Autodesk Inventor part; units mm, degrees
(part 3 of 3)
  line L755 (119.1, 110.9) -> (119.1, 119.1)
  line L756 (110.9, 100.9) -> (119.1, 100.9)
  line L757 (119.1, 119.1) -> (110.9, 119.1)
  line L758 (110.9, 119.1) -> (110.9, 120.9) construction
  line L759 (110.9, 120.9) -> (119.1, 120.9)
  line L760 (119.1, 120.9) -> (119.1, 129.1)
  line L761 (110.9, 129.1) -> (110.9, 120.9)
  line L762 (119.1, 139.1) -> (110.9, 139.1)
  line L763 (110.9, 140.9) -> (110.9, 139.1) construction
  line L764 (110.9, 130.9) -> (119.1, 130.9)
  line L765 (110.9, 139.1) -> (110.9, 130.9)
  line L766 (119.1, 129.1) -> (110.9, 129.1)
  line L767 (110.9, 129.1) -> (110.9, 130.9) construction
  line L768 (119.1, 130.9) -> (119.1, 139.1)
  line L769 (119.1, 160.9) -> (119.1, 169.1)
  line L770 (110.9, 169.1) -> (110.9, 160.9)
  line L771 (119.1, 169.1) -> (110.9, 169.1)
  line L772 (110.9, 169.1) -> (110.9, 170.9) construction
  line L773 (110.9, 170.9) -> (119.1, 170.9)
  line L774 (110.9, 179.1) -> (110.9, 170.9)
  line L775 (119.1, 170.9) -> (119.1, 179.1)
  line L776 (119.1, 179.1) -> (110.9, 179.1)
  line L777 (119.1, 149.1) -> (110.9, 149.1)
  line L778 (119.1, 140.9) -> (119.1, 149.1)
  line L779 (110.9, 150.9) -> (119.1, 150.9)
  line L780 (110.9, 149.1) -> (110.9, 150.9) construction
  line L781 (119.1, 150.9) -> (119.1, 159.1)
  line L782 (119.1, 159.1) -> (110.9, 159.1)
  line L783 (110.9, 159.1) -> (110.9, 150.9)
  line L784 (110.9, 160.9) -> (119.1, 160.9)
  line L785 (110.9, 159.1) -> (110.9, 160.9) construction
  line L786 (110.9, 149.1) -> (110.9, 140.9)
  line L787 (110.9, 140.9) -> (119.1, 140.9)
  line L788 (119.1, 60.9) -> (119.1, 69.1)
  line L789 (110.9, 69.1) -> (110.9, 60.9)
  line L790 (119.1, 69.1) -> (110.9, 69.1)
  line L791 (110.9, 69.1) -> (110.9, 70.9) construction
  line L792 (110.9, 70.9) -> (119.1, 70.9)
  line L793 (119.1, 70.9) -> (119.1, 79.1)
  line L794 (110.9, 79.1) -> (110.9, 70.9)
  line L795 (119.1, 79.1) -> (110.9, 79.1)
  line L796 (110.9, 79.1) -> (110.9, 80.9) construction
  line L797 (119.1, 80.9) -> (119.1, 89.1)
  line L798 (110.9, 89.1) -> (110.9, 80.9)
  line L799 (110.9, 80.9) -> (119.1, 80.9)
  line L800 (109.1, 20.9) -> (110.9, 20.9) construction
  line L801 (120.9, 20.9) -> (129.1, 20.9)
  line L802 (129.1, 20.9) -> (129.1, 29.1)
  line L803 (129.1, 29.1) -> (120.9, 29.1)
  line L804 (120.9, 29.1) -> (120.9, 20.9)
  line L805 (130.9, 20.9) -> (139.1, 20.9)
  line L806 (139.1, 20.9) -> (139.1, 29.1)
  line L807 (130.9, 29.1) -> (130.9, 20.9)
  line L808 (129.1, 20.9) -> (130.9, 20.9) construction
  line L809 (129.1, 89.1) -> (120.9, 89.1)
  line L810 (120.9, 90.9) -> (129.1, 90.9)
  line L811 (120.9, 89.1) -> (120.9, 90.9) construction
  line L812 (129.1, 90.9) -> (129.1, 99.1)
  line L813 (139.1, 90.9) -> (139.1, 99.1)
  line L814 (130.9, 90.9) -> (139.1, 90.9)
  line L815 (139.1, 89.1) -> (130.9, 89.1)
  line L816 (130.9, 99.1) -> (130.9, 90.9)
  line L817 (130.9, 89.1) -> (130.9, 90.9) construction
  line L818 (129.1, 99.1) -> (120.9, 99.1)
  line L819 (120.9, 100.9) -> (129.1, 100.9)
  line L820 (120.9, 99.1) -> (120.9, 100.9) construction
  line L821 (120.9, 99.1) -> (120.9, 90.9)
  line L822 (129.1, 59.1) -> (120.9, 59.1)
  line L823 (139.1, 59.1) -> (130.9, 59.1)
  line L824 (130.9, 60.9) -> (130.9, 59.1) construction
  line L825 (130.9, 60.9) -> (139.1, 60.9)
  line L826 (139.1, 60.9) -> (139.1, 69.1)
  line L827 (120.9, 60.9) -> (120.9, 59.1) construction
  line L828 (120.9, 60.9) -> (129.1, 60.9)
  line L829 (130.9, 69.1) -> (130.9, 60.9)
  line L830 (129.1, 60.9) -> (129.1, 69.1)
  line L831 (120.9, 69.1) -> (120.9, 60.9)
  line L832 (129.1, 69.1) -> (120.9, 69.1)
  line L833 (120.9, 70.9) -> (129.1, 70.9)
  line L834 (120.9, 69.1) -> (120.9, 70.9) construction
  line L835 (120.9, 140.9) -> (129.1, 140.9)
  line L836 (120.9, 140.9) -> (120.9, 139.1) construction
  line L837 (130.9, 139.1) -> (130.9, 130.9)
  line L838 (129.1, 139.1) -> (120.9, 139.1)
  line L839 (129.1, 130.9) -> (129.1, 139.1)
  line L840 (130.9, 129.1) -> (130.9, 130.9) construction
  line L841 (120.9, 139.1) -> (120.9, 130.9)
  line L842 (120.9, 130.9) -> (129.1, 130.9)
  line L843 (120.9, 129.1) -> (120.9, 130.9) construction
  line L844 (129.1, 129.1) -> (120.9, 129.1)
  line L845 (130.9, 140.9) -> (130.9, 139.1) construction
  line L846 (130.9, 130.9) -> (139.1, 130.9)
  line L847 (139.1, 130.9) -> (139.1, 139.1)
  line L848 (120.9, 149.1) -> (120.9, 140.9)
  line L849 (139.1, 139.1) -> (130.9, 139.1)
  line L850 (129.1, 140.9) -> (129.1, 149.1)
  line L851 (130.9, 140.9) -> (139.1, 140.9)
  line L852 (130.9, 149.1) -> (130.9, 140.9)
  line L853 (139.1, 140.9) -> (139.1, 149.1)
  line L854 (120.9, 30.9) -> (129.1, 30.9)
  line L855 (129.1, 30.9) -> (129.1, 39.1)
  line L856 (129.1, 39.1) -> (120.9, 39.1)
  line L857 (120.9, 39.1) -> (120.9, 30.9)
  line L858 (120.9, 29.1) -> (120.9, 30.9) construction
  line L859 (130.9, 29.1) -> (130.9, 30.9) construction
  line L860 (120.9, 40.9) -> (129.1, 40.9)
  line L861 (120.9, 39.1) -> (120.9, 40.9) construction
  line L862 (139.1, 29.1) -> (130.9, 29.1)
  line L863 (130.9, 39.1) -> (130.9, 30.9)
  line L864 (130.9, 30.9) -> (139.1, 30.9)
  line L865 (130.9, 39.1) -> (130.9, 40.9) construction
  line L866 (139.1, 30.9) -> (139.1, 39.1)
  line L867 (139.1, 39.1) -> (130.9, 39.1)
  line L868 (130.9, 40.9) -> (139.1, 40.9)
  line L869 (129.1, 40.9) -> (129.1, 49.1)
  line L870 (129.1, 49.1) -> (120.9, 49.1)
  line L871 (120.9, 49.1) -> (120.9, 40.9)
  line L872 (120.9, 50.9) -> (129.1, 50.9)
  line L873 (129.1, 50.9) -> (129.1, 59.1)
  line L874 (120.9, 59.1) -> (120.9, 50.9)
  line L875 (120.9, 49.1) -> (120.9, 50.9) construction
  line L876 (130.9, 59.1) -> (130.9, 50.9)
  line L877 (139.1, 50.9) -> (139.1, 59.1)
  line L878 (130.9, 49.1) -> (130.9, 50.9) construction
  line L879 (130.9, 50.9) -> (139.1, 50.9)
  line L880 (139.1, 49.1) -> (130.9, 49.1)
  line L881 (130.9, 49.1) -> (130.9, 40.9)
  line L882 (139.1, 40.9) -> (139.1, 49.1)
  line L883 (139.1, 109.1) -> (130.9, 109.1)
  line L884 (130.9, 109.1) -> (130.9, 110.9) construction
  line L885 (130.9, 110.9) -> (139.1, 110.9)
  line L886 (139.1, 119.1) -> (130.9, 119.1)
  line L887 (130.9, 119.1) -> (130.9, 110.9)
  line L888 (130.9, 119.1) -> (130.9, 120.9) construction
  line L889 (130.9, 120.9) -> (139.1, 120.9)
  line L890 (139.1, 110.9) -> (139.1, 119.1)
  line L891 (129.1, 110.9) -> (129.1, 119.1)
  line L892 (120.9, 119.1) -> (120.9, 110.9)
  line L893 (129.1, 119.1) -> (120.9, 119.1)
  line L894 (120.9, 119.1) -> (120.9, 120.9) construction
  line L895 (120.9, 120.9) -> (129.1, 120.9)
  line L896 (129.1, 120.9) -> (129.1, 129.1)
  line L897 (120.9, 129.1) -> (120.9, 120.9)
  line L898 (130.9, 129.1) -> (130.9, 120.9)
  line L899 (139.1, 120.9) -> (139.1, 129.1)
  line L900 (139.1, 129.1) -> (130.9, 129.1)
  line L901 (129.1, 149.1) -> (120.9, 149.1)
  line L902 (120.9, 149.1) -> (120.9, 150.9) construction
  line L903 (120.9, 150.9) -> (129.1, 150.9)
  line L904 (129.1, 159.1) -> (120.9, 159.1)
  line L905 (129.1, 150.9) -> (129.1, 159.1)
  line L906 (120.9, 159.1) -> (120.9, 150.9)
  line L907 (120.9, 159.1) -> (120.9, 160.9) construction
  line L908 (120.9, 160.9) -> (129.1, 160.9)
  line L909 (130.9, 150.9) -> (139.1, 150.9)
  line L910 (130.9, 149.1) -> (130.9, 150.9) construction
  line L911 (130.9, 159.1) -> (130.9, 150.9)
  line L912 (130.9, 159.1) -> (130.9, 160.9) construction
  line L913 (139.1, 159.1) -> (130.9, 159.1)
  line L914 (139.1, 150.9) -> (139.1, 159.1)
  line L915 (130.9, 160.9) -> (139.1, 160.9)
  line L916 (139.1, 149.1) -> (130.9, 149.1)
  line L917 (130.9, 99.1) -> (130.9, 100.9) construction
  line L918 (129.1, 109.1) -> (120.9, 109.1)
  line L919 (120.9, 109.1) -> (120.9, 100.9)
  line L920 (120.9, 110.9) -> (129.1, 110.9)
  line L921 (120.9, 109.1) -> (120.9, 110.9) construction
  line L922 (129.1, 100.9) -> (129.1, 109.1)
  line L923 (139.1, 99.1) -> (130.9, 99.1)
  line L924 (130.9, 109.1) -> (130.9, 100.9)
  line L925 (139.1, 100.9) -> (139.1, 109.1)
  line L926 (130.9, 100.9) -> (139.1, 100.9)
  line L927 (129.1, 79.1) -> (120.9, 79.1)
  line L928 (120.9, 79.1) -> (120.9, 80.9) construction
  line L929 (120.9, 80.9) -> (129.1, 80.9)
  line L930 (129.1, 80.9) -> (129.1, 89.1)
  line L931 (120.9, 89.1) -> (120.9, 80.9)
  line L932 (129.1, 70.9) -> (129.1, 79.1)
  line L933 (120.9, 79.1) -> (120.9, 70.9)
  line L934 (139.1, 69.1) -> (130.9, 69.1)
  line L935 (130.9, 69.1) -> (130.9, 70.9) construction
  line L936 (130.9, 70.9) -> (139.1, 70.9)
  line L937 (139.1, 70.9) -> (139.1, 79.1)
  line L938 (130.9, 79.1) -> (130.9, 70.9)
  line L939 (139.1, 79.1) -> (130.9, 79.1)
  line L940 (130.9, 79.1) -> (130.9, 80.9) construction
  line L941 (130.9, 80.9) -> (139.1, 80.9)
  line L942 (130.9, 89.1) -> (130.9, 80.9)
  line L943 (139.1, 80.9) -> (139.1, 89.1)
  line L944 (129.1, 160.9) -> (129.1, 169.1)
  line L945 (129.1, 169.1) -> (120.9, 169.1)
  line L946 (120.9, 169.1) -> (120.9, 160.9)
  line L947 (120.9, 170.9) -> (129.1, 170.9)
  line L948 (120.9, 169.1) -> (120.9, 170.9) construction
  line L949 (129.1, 170.9) -> (129.1, 179.1)
  line L950 (129.1, 179.1) -> (120.9, 179.1)
  line L951 (120.9, 179.1) -> (120.9, 170.9)
  line L952 (139.1, 160.9) -> (139.1, 169.1)
  line L953 (130.9, 169.1) -> (130.9, 160.9)
  line L954 (139.1, 169.1) -> (130.9, 169.1)
  line L955 (130.9, 169.1) -> (130.9, 170.9) construction
  line L956 (130.9, 179.1) -> (130.9, 170.9)
  line L957 (139.1, 170.9) -> (139.1, 179.1)
  line L958 (139.1, 179.1) -> (130.9, 179.1)
  line L959 (130.9, 170.9) -> (139.1, 170.9)
  line L960 (119.1, 20.9) -> (120.9, 20.9) construction
  line L961 (159.1, 20.9) -> (160.9, 20.9) construction
  line L962 (160.9, 29.1) -> (160.9, 20.9)
  line L963 (169.1, 29.1) -> (160.9, 29.1)
  line L964 (160.9, 20.9) -> (169.1, 20.9)
  line L965 (169.1, 20.9) -> (169.1, 29.1)
  line L966 (169.1, 20.9) -> (170.9, 20.9) construction
  line L967 (170.9, 29.1) -> (170.9, 20.9)
  line L968 (170.9, 20.9) -> (179.1, 20.9)
  line L969 (179.1, 20.9) -> (179.1, 29.1)
  line L970 (159.1, 20.9) -> (159.1, 29.1)
  line L971 (149.1, 39.1) -> (140.9, 39.1)
  line L972 (140.9, 40.9) -> (149.1, 40.9)
  line L973 (149.1, 40.9) -> (149.1, 49.1)
  line L974 (149.1, 49.1) -> (140.9, 49.1)
  line L975 (140.9, 49.1) -> (140.9, 40.9)
  line L976 (140.9, 50.9) -> (149.1, 50.9)
  line L977 (150.9, 49.1) -> (150.9, 50.9) construction
  line L978 (140.9, 39.1) -> (140.9, 40.9) construction
  line L979 (150.9, 50.9) -> (159.1, 50.9)
  line L980 (150.9, 49.1) -> (150.9, 40.9)
  line L981 (150.9, 39.1) -> (150.9, 40.9) construction
  line L982 (150.9, 40.9) -> (159.1, 40.9)
  line L983 (159.1, 40.9) -> (159.1, 49.1)
  line L984 (159.1, 39.1) -> (150.9, 39.1)
  line L985 (159.1, 49.1) -> (150.9, 49.1)
  line L986 (149.1, 20.9) -> (149.1, 29.1)
  line L987 (150.9, 29.1) -> (150.9, 20.9)
  line L988 (150.9, 20.9) -> (159.1, 20.9)
  line L989 (149.1, 20.9) -> (150.9, 20.9) construction
  line L990 (159.1, 30.9) -> (159.1, 39.1)
  line L991 (159.1, 29.1) -> (150.9, 29.1)
  line L992 (150.9, 30.9) -> (159.1, 30.9)
  line L993 (150.9, 29.1) -> (150.9, 30.9) construction
  line L994 (150.9, 39.1) -> (150.9, 30.9)
  line L995 (149.1, 30.9) -> (149.1, 39.1)
  line L996 (149.1, 79.1) -> (140.9, 79.1)
  line L997 (140.9, 79.1) -> (140.9, 80.9) construction
  line L998 (140.9, 80.9) -> (149.1, 80.9)
  line L999 (150.9, 79.1) -> (150.9, 80.9) construction
  line L1000 (149.1, 89.1) -> (140.9, 89.1)
  line L1001 (140.9, 89.1) -> (140.9, 80.9)
  line L1002 (149.1, 80.9) -> (149.1, 89.1)
  line L1003 (149.1, 99.1) -> (140.9, 99.1)
  line L1004 (140.9, 99.1) -> (140.9, 100.9) construction
  line L1005 (140.9, 100.9) -> (149.1, 100.9)
  line L1006 (140.9, 109.1) -> (140.9, 100.9)
  line L1007 (149.1, 109.1) -> (140.9, 109.1)
  line L1008 (140.9, 110.9) -> (149.1, 110.9)
  line L1009 (140.9, 109.1) -> (140.9, 110.9) construction
  line L1010 (150.9, 80.9) -> (159.1, 80.9)
  line L1011 (150.9, 79.1) -> (150.9, 70.9)
  line L1012 (159.1, 79.1) -> (150.9, 79.1)
  line L1013 (149.1, 70.9) -> (149.1, 79.1)
  line L1014 (140.9, 79.1) -> (140.9, 70.9)
  line L1015 (159.1, 70.9) -> (159.1, 79.1)
  line L1016 (140.9, 70.9) -> (149.1, 70.9)
  line L1017 (150.9, 69.1) -> (150.9, 70.9) construction
  line L1018 (149.1, 69.1) -> (140.9, 69.1)
  line L1019 (140.9, 69.1) -> (140.9, 70.9) construction
  line L1020 (150.9, 70.9) -> (159.1, 70.9)
  line L1021 (159.1, 69.1) -> (150.9, 69.1)
  line L1022 (159.1, 60.9) -> (159.1, 69.1)
  line L1023 (150.9, 69.1) -> (150.9, 60.9)
  line L1024 (149.1, 60.9) -> (149.1, 69.1)
  line L1025 (140.9, 60.9) -> (149.1, 60.9)
  line L1026 (140.9, 69.1) -> (140.9, 60.9)
  line L1027 (149.1, 119.1) -> (140.9, 119.1)
  line L1028 (140.9, 119.1) -> (140.9, 120.9) construction
  line L1029 (140.9, 120.9) -> (149.1, 120.9)
  line L1030 (149.1, 120.9) -> (149.1, 129.1)
  line L1031 (140.9, 129.1) -> (140.9, 120.9)
  line L1032 (149.1, 129.1) -> (140.9, 129.1)
  line L1033 (140.9, 140.9) -> (149.1, 140.9)
  line L1034 (149.1, 139.1) -> (140.9, 139.1)
  line L1035 (140.9, 140.9) -> (140.9, 139.1) construction
  line L1036 (149.1, 130.9) -> (149.1, 139.1)
  line L1037 (140.9, 130.9) -> (149.1, 130.9)
  line L1038 (140.9, 139.1) -> (140.9, 130.9)
  line L1039 (140.9, 129.1) -> (140.9, 130.9) construction
  line L1040 (140.9, 159.1) -> (140.9, 160.9) construction
  line L1041 (140.9, 160.9) -> (149.1, 160.9)
  line L1042 (149.1, 159.1) -> (140.9, 159.1)
  line L1043 (140.9, 150.9) -> (149.1, 150.9)
  line L1044 (149.1, 149.1) -> (140.9, 149.1)
  line L1045 (140.9, 149.1) -> (140.9, 150.9) construction
  line L1046 (140.9, 159.1) -> (140.9, 150.9)
  line L1047 (149.1, 150.9) -> (149.1, 159.1)
  line L1048 (140.9, 169.1) -> (140.9, 160.9)
  line L1049 (150.9, 179.1) -> (150.9, 170.9)
  line L1050 (149.1, 169.1) -> (140.9, 169.1)
  line L1051 (140.9, 169.1) -> (140.9, 170.9) construction
  line L1052 (140.9, 170.9) -> (149.1, 170.9)
  line L1053 (140.9, 179.1) -> (140.9, 170.9)
  line L1054 (149.1, 179.1) -> (140.9, 179.1)
  line L1055 (149.1, 170.9) -> (149.1, 179.1)
  line L1056 (149.1, 50.9) -> (149.1, 59.1)
  line L1057 (149.1, 59.1) -> (140.9, 59.1)
  line L1058 (160.9, 59.1) -> (160.9, 50.9)
  line L1059 (159.1, 50.9) -> (159.1, 59.1)
  line L1060 (159.1, 59.1) -> (150.9, 59.1)
  line L1061 (160.9, 60.9) -> (160.9, 59.1) construction
  line L1062 (150.9, 60.9) -> (159.1, 60.9)
  line L1063 (150.9, 59.1) -> (150.9, 50.9)
  line L1064 (150.9, 60.9) -> (150.9, 59.1) construction
  line L1065 (140.9, 49.1) -> (140.9, 50.9) construction
  line L1066 (140.9, 60.9) -> (140.9, 59.1) construction
  line L1067 (140.9, 59.1) -> (140.9, 50.9)
  line L1068 (140.9, 90.9) -> (149.1, 90.9)
  line L1069 (140.9, 99.1) -> (140.9, 90.9)
  line L1070 (140.9, 89.1) -> (140.9, 90.9) construction
  line L1071 (149.1, 90.9) -> (149.1, 99.1)
  line L1072 (159.1, 99.1) -> (150.9, 99.1)
  line L1073 (150.9, 99.1) -> (150.9, 90.9)
  line L1074 (150.9, 89.1) -> (150.9, 90.9) construction
  line L1075 (150.9, 90.9) -> (159.1, 90.9)
  line L1076 (159.1, 89.1) -> (150.9, 89.1)
  line L1077 (159.1, 90.9) -> (159.1, 99.1)
  line L1078 (149.1, 110.9) -> (149.1, 119.1)
  line L1079 (140.9, 119.1) -> (140.9, 110.9)
  line L1080 (149.1, 100.9) -> (149.1, 109.1)
  line L1081 (150.9, 99.1) -> (150.9, 100.9) construction
  line L1082 (160.9, 99.1) -> (160.9, 100.9) construction
  line L1083 (169.1, 99.1) -> (160.9, 99.1)
  line L1084 (159.1, 100.9) -> (159.1, 109.1)
  line L1085 (150.9, 109.1) -> (150.9, 100.9)
  line L1086 (159.1, 109.1) -> (150.9, 109.1)
  line L1087 (160.9, 100.9) -> (169.1, 100.9)
  line L1088 (150.9, 109.1) -> (150.9, 110.9) construction
  line L1089 (160.9, 109.1) -> (160.9, 100.9)
  line L1090 (150.9, 110.9) -> (159.1, 110.9)
  line L1091 (160.9, 109.1) -> (160.9, 110.9) construction
  line L1092 (169.1, 109.1) -> (160.9, 109.1)
  line L1093 (160.9, 110.9) -> (169.1, 110.9)
  line L1094 (150.9, 119.1) -> (150.9, 110.9)
  line L1095 (150.9, 100.9) -> (159.1, 100.9)
  line L1096 (160.9, 130.9) -> (169.1, 130.9)
  line L1097 (169.1, 129.1) -> (160.9, 129.1)
  line L1098 (160.9, 139.1) -> (160.9, 130.9)
  line L1099 (160.9, 129.1) -> (160.9, 130.9) construction
  line L1100 (159.1, 130.9) -> (159.1, 139.1)
  line L1101 (150.9, 140.9) -> (150.9, 139.1) construction
  line L1102 (159.1, 139.1) -> (150.9, 139.1)
  line L1103 (150.9, 139.1) -> (150.9, 130.9)
  line L1104 (159.1, 120.9) -> (159.1, 129.1)
  line L1105 (150.9, 130.9) -> (159.1, 130.9)
  line L1106 (150.9, 129.1) -> (150.9, 130.9) construction
  line L1107 (159.1, 129.1) -> (150.9, 129.1)
  line L1108 (150.9, 129.1) -> (150.9, 120.9)
  line L1109 (150.9, 120.9) -> (159.1, 120.9)
  line L1110 (159.1, 119.1) -> (150.9, 119.1)
  line L1111 (150.9, 119.1) -> (150.9, 120.9) construction
  line L1112 (169.1, 130.9) -> (169.1, 139.1)
  line L1113 (170.9, 139.1) -> (170.9, 130.9)
  line L1114 (179.1, 130.9) -> (179.1, 139.1)
  line L1115 (159.1, 170.9) -> (159.1, 179.1)
  line L1116 (159.1, 179.1) -> (150.9, 179.1)
  line L1117 (160.9, 179.1) -> (160.9, 170.9)
  line L1118 (149.1, 160.9) -> (149.1, 169.1)
  line L1119 (150.9, 170.9) -> (159.1, 170.9)
  line L1120 (150.9, 169.1) -> (150.9, 160.9)
  line L1121 (159.1, 169.1) -> (150.9, 169.1)
  line L1122 (160.9, 169.1) -> (160.9, 170.9) construction
  line L1123 (159.1, 160.9) -> (159.1, 169.1)
  line L1124 (150.9, 169.1) -> (150.9, 170.9) construction
  line L1125 (140.9, 149.1) -> (140.9, 140.9)
  line L1126 (149.1, 140.9) -> (149.1, 149.1)
  line L1127 (150.9, 140.9) -> (159.1, 140.9)
  line L1128 (150.9, 149.1) -> (150.9, 140.9)
  line L1129 (159.1, 140.9) -> (159.1, 149.1)
  line L1130 (150.9, 149.1) -> (150.9, 150.9) construction
  line L1131 (159.1, 149.1) -> (150.9, 149.1)
  line L1132 (150.9, 159.1) -> (150.9, 150.9)
  line L1133 (150.9, 159.1) -> (150.9, 160.9) construction
  line L1134 (159.1, 150.9) -> (159.1, 159.1)
  line L1135 (159.1, 159.1) -> (150.9, 159.1)
  line L1136 (150.9, 160.9) -> (159.1, 160.9)
  line L1137 (150.9, 150.9) -> (159.1, 150.9)
  line L1138 (140.9, 20.9) -> (149.1, 20.9)
  line L1139 (149.1, 29.1) -> (140.9, 29.1)
  line L1140 (140.9, 29.1) -> (140.9, 20.9)
  line L1141 (140.9, 30.9) -> (149.1, 30.9)
  line L1142 (140.9, 39.1) -> (140.9, 30.9)
  line L1143 (140.9, 29.1) -> (140.9, 30.9) construction
  line L1144 (169.1, 100.9) -> (169.1, 109.1)
  line L1145 (170.9, 109.1) -> (170.9, 100.9)
  line L1146 (170.9, 99.1) -> (170.9, 100.9) construction
  line L1147 (179.1, 100.9) -> (179.1, 109.1)
  line L1148 (170.9, 100.9) -> (179.1, 100.9)
  line L1149 (179.1, 99.1) -> (170.9, 99.1)
  line L1150 (159.1, 110.9) -> (159.1, 119.1)
  line L1151 (160.9, 119.1) -> (160.9, 110.9)
  line L1152 (179.1, 109.1) -> (170.9, 109.1)
  line L1153 (169.1, 110.9) -> (169.1, 119.1)
  line L1154 (170.9, 110.9) -> (179.1, 110.9)
  line L1155 (170.9, 119.1) -> (170.9, 110.9)
  line L1156 (179.1, 110.9) -> (179.1, 119.1)
  line L1157 (179.1, 119.1) -> (170.9, 119.1)
  line L1158 (170.9, 109.1) -> (170.9, 110.9) construction
  line L1159 (170.9, 149.1) -> (170.9, 150.9) construction
  line L1160 (179.1, 150.9) -> (179.1, 159.1)
  line L1161 (169.1, 149.1) -> (160.9, 149.1)
  line L1162 (160.9, 149.1) -> (160.9, 150.9) construction
  line L1163 (160.9, 150.9) -> (169.1, 150.9)
  line L1164 (169.1, 150.9) -> (169.1, 159.1)
  line L1165 (160.9, 159.1) -> (160.9, 150.9)
  line L1166 (170.9, 159.1) -> (170.9, 150.9)
  line L1167 (160.9, 149.1) -> (160.9, 140.9)
  line L1168 (160.9, 140.9) -> (160.9, 139.1) construction
  line L1169 (160.9, 140.9) -> (169.1, 140.9)
  line L1170 (169.1, 140.9) -> (169.1, 149.1)
  line L1171 (170.9, 149.1) -> (170.9, 140.9)
  line L1172 (170.9, 140.9) -> (170.9, 139.1) construction
  line L1173 (170.9, 150.9) -> (179.1, 150.9)
  line L1174 (179.1, 149.1) -> (170.9, 149.1)
  line L1175 (179.1, 140.9) -> (179.1, 149.1)
  line L1176 (170.9, 140.9) -> (179.1, 140.9)
  line L1177 (179.1, 139.1) -> (170.9, 139.1)
  line L1178 (169.1, 139.1) -> (160.9, 139.1)
  line L1179 (160.9, 29.1) -> (160.9, 30.9) construction
  line L1180 (160.9, 30.9) -> (169.1, 30.9)
  line L1181 (170.9, 29.1) -> (170.9, 30.9) construction
  line L1182 (179.1, 29.1) -> (170.9, 29.1)
  line L1183 (169.1, 30.9) -> (169.1, 39.1)
  line L1184 (169.1, 39.1) -> (160.9, 39.1)
  line L1185 (160.9, 39.1) -> (160.9, 30.9)
  line L1186 (170.9, 39.1) -> (170.9, 30.9)
  line L1187 (170.9, 30.9) -> (179.1, 30.9)
  line L1188 (179.1, 30.9) -> (179.1, 39.1)
  line L1189 (160.9, 39.1) -> (160.9, 40.9) construction
  line L1190 (160.9, 40.9) -> (169.1, 40.9)
  line L1191 (170.9, 39.1) -> (170.9, 40.9) construction
  line L1192 (160.9, 49.1) -> (160.9, 40.9)
  line L1193 (179.1, 39.1) -> (170.9, 39.1)
  line L1194 (170.9, 40.9) -> (179.1, 40.9)
  line L1195 (169.1, 40.9) -> (169.1, 49.1)
  line L1196 (170.9, 49.1) -> (170.9, 40.9)
  line L1197 (179.1, 40.9) -> (179.1, 49.1)
  line L1198 (170.9, 60.9) -> (179.1, 60.9)
  line L1199 (179.1, 60.9) -> (179.1, 69.1)
  line L1200 (160.9, 60.9) -> (169.1, 60.9)
  line L1201 (170.9, 69.1) -> (170.9, 60.9)
  line L1202 (169.1, 60.9) -> (169.1, 69.1)
  line L1203 (160.9, 69.1) -> (160.9, 60.9)
  line L1204 (169.1, 69.1) -> (160.9, 69.1)
  line L1205 (160.9, 70.9) -> (169.1, 70.9)
  line L1206 (160.9, 69.1) -> (160.9, 70.9) construction
  line L1207 (170.9, 69.1) -> (170.9, 70.9) construction
  line L1208 (170.9, 70.9) -> (179.1, 70.9)
  line L1209 (160.9, 79.1) -> (160.9, 70.9)
  line L1210 (169.1, 70.9) -> (169.1, 79.1)
  line L1211 (170.9, 79.1) -> (170.9, 70.9)
  line L1212 (179.1, 70.9) -> (179.1, 79.1)
  line L1213 (179.1, 69.1) -> (170.9, 69.1)
  line L1214 (169.1, 89.1) -> (160.9, 89.1)
  line L1215 (160.9, 90.9) -> (169.1, 90.9)
  line L1216 (160.9, 89.1) -> (160.9, 90.9) construction
  line L1217 (169.1, 90.9) -> (169.1, 99.1)
  line L1218 (179.1, 90.9) -> (179.1, 99.1)
  line L1219 (170.9, 90.9) -> (179.1, 90.9)
  line L1220 (179.1, 89.1) -> (170.9, 89.1)
  line L1221 (170.9, 99.1) -> (170.9, 90.9)
  line L1222 (170.9, 89.1) -> (170.9, 90.9) construction
  line L1223 (160.9, 99.1) -> (160.9, 90.9)
  line L1224 (160.9, 80.9) -> (169.1, 80.9)
  line L1225 (160.9, 89.1) -> (160.9, 80.9)
  line L1226 (169.1, 79.1) -> (160.9, 79.1)
  line L1227 (160.9, 79.1) -> (160.9, 80.9) construction
  line L1228 (169.1, 80.9) -> (169.1, 89.1)
  line L1229 (170.9, 89.1) -> (170.9, 80.9)
  line L1230 (179.1, 80.9) -> (179.1, 89.1)
  line L1231 (179.1, 79.1) -> (170.9, 79.1)
  line L1232 (170.9, 80.9) -> (179.1, 80.9)
  line L1233 (169.1, 159.1) -> (160.9, 159.1)
  line L1234 (179.1, 159.1) -> (170.9, 159.1)
  line L1235 (160.9, 159.1) -> (160.9, 160.9) construction
  line L1236 (170.9, 159.1) -> (170.9, 160.9) construction
  line L1237 (160.9, 160.9) -> (169.1, 160.9)
  line L1238 (170.9, 160.9) -> (179.1, 160.9)
  line L1239 (160.9, 169.1) -> (160.9, 160.9)
  line L1240 (169.1, 169.1) -> (160.9, 169.1)
  line L1241 (169.1, 160.9) -> (169.1, 169.1)
  line L1242 (170.9, 169.1) -> (170.9, 160.9)
  line L1243 (179.1, 160.9) -> (179.1, 169.1)
  line L1244 (160.9, 49.1) -> (160.9, 50.9) construction
  line L1245 (169.1, 59.1) -> (160.9, 59.1)
  line L1246 (169.1, 50.9) -> (169.1, 59.1)
  line L1247 (170.9, 60.9) -> (170.9, 59.1) construction
  line L1248 (169.1, 49.1) -> (160.9, 49.1)
  line L1249 (170.9, 59.1) -> (170.9, 50.9)
  line L1250 (170.9, 49.1) -> (170.9, 50.9) construction
  line L1251 (179.1, 59.1) -> (170.9, 59.1)
  line L1252 (179.1, 50.9) -> (179.1, 59.1)
  line L1253 (170.9, 50.9) -> (179.1, 50.9)
  line L1254 (179.1, 49.1) -> (170.9, 49.1)
  line L1255 (160.9, 50.9) -> (169.1, 50.9)
  line L1256 (170.9, 129.1) -> (170.9, 130.9) construction
  line L1257 (160.9, 129.1) -> (160.9, 120.9)
  line L1258 (160.9, 120.9) -> (169.1, 120.9)
  line L1259 (160.9, 119.1) -> (160.9, 120.9) construction
  line L1260 (169.1, 119.1) -> (160.9, 119.1)
  line L1261 (169.1, 120.9) -> (169.1, 129.1)
  line L1262 (170.9, 130.9) -> (179.1, 130.9)
  line L1263 (170.9, 129.1) -> (170.9, 120.9)
  line L1264 (179.1, 129.1) -> (170.9, 129.1)
  line L1265 (170.9, 119.1) -> (170.9, 120.9) construction
  line L1266 (170.9, 120.9) -> (179.1, 120.9)
  line L1267 (179.1, 120.9) -> (179.1, 129.1)
  line L1268 (160.9, 170.9) -> (169.1, 170.9)
  line L1269 (169.1, 179.1) -> (160.9, 179.1)
  line L1270 (169.1, 170.9) -> (169.1, 179.1)
  line L1271 (170.9, 169.1) -> (170.9, 170.9) construction
  line L1272 (170.9, 179.1) -> (170.9, 170.9)
  line L1273 (179.1, 170.9) -> (179.1, 179.1)
  line L1274 (179.1, 179.1) -> (170.9, 179.1)
  line L1275 (170.9, 170.9) -> (179.1, 170.9)
  line L1276 (179.1, 169.1) -> (170.9, 169.1)
  line L1277 (150.9, 89.1) -> (150.9, 80.9)
  line L1278 (159.1, 80.9) -> (159.1, 89.1)
  line L1279 (170.9, 79.1) -> (170.9, 80.9) construction
  line L1280 (139.1, 20.9) -> (140.9, 20.9) construction
  line L1281 (99.1, 20.9) -> (100.9, 20.9) construction
  line L1282 (10, 21.9) -> (20, 21.9) construction
  line L1283 (21.9, 10) -> (178.1, 10) projected
  line L1284 (21.9, 0) -> (21.9, 10) projected
  line L1285 (0, 0) -> (21.9, 0) projected
  line L1286 (0, 21.9) -> (0, 0) projected
  line L1287 (10, 21.9) -> (0, 21.9) projected
  line L1288 (10, 178.1) -> (10, 21.9) projected
  line L1289 (0, 178.1) -> (10, 178.1) projected
  line L1290 (0, 200) -> (0, 178.1) projected
  line L1291 (21.9, 200) -> (0, 200) projected
  line L1292 (21.9, 190) -> (21.9, 200) projected
  line L1293 (178.1, 190) -> (21.9, 190) projected
  line L1294 (200, 200) -> (178.1, 200) projected
  line L1295 (178.1, 200) -> (178.1, 190) projected
  line L1296 (200, 178.1) -> (200, 200) projected
  line L1297 (190, 178.1) -> (200, 178.1) projected
  line L1298 (190, 21.9) -> (190, 178.1) projected
  line L1299 (200, 21.9) -> (190, 21.9) projected
  line L1300 (200, 0) -> (200, 21.9) projected
  line L1301 (178.1, 0) -> (200, 0) projected
  line L1302 (178.1, 10) -> (178.1, 0) projected
  dimension "d26" = 1.8
  dimension "d27" = 8.2
  dimension "d29" = 1
  constraints: 2564 end point, 766 equal length, 512 parallel, 272 horizontal, 258 perpendicular, 162 point on line, 80 vertical
  measures "d26" distance of L2.end L4.start
  measures "d27" distance of L2.end L0.start
  measures "d29" distance of L19.start L19.end
extrude "Extrusion4" add sketch "Skizze2" along normal blind 3
